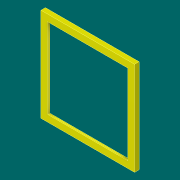
# Autodesk Inventor part: mirrorFrontFrame
Saved by Autodesk Inventor 2016 (Build 200138000, 138)
## iProperties
Created: 2015-10-27
Part Number: mirrorFrontFrame
Material: ABS Plastic
Document SubType Name: Modeling
Designer: Sawaiz
Density: 1.06 g/cm^3
Appearance: Smooth - Yellow
Author: Sawaiz
Autodesk Inventor part; units mm, degrees
ref_plane "YZ Plane" through (0, 0, 0) normal (1, 0, 0) x (0, 1, 0)
ref_plane "XZ Plane" through (0, 0, 0) normal (0, 1, 0) x (-1, 0, 0)
ref_plane "XY Plane" through (0, 0, 0) normal (0, 0, 1) x (1, 0, 0)
sketch "Sketch1" plane through (0, 0, 0) normal (1, 0, 0) x (0, 1, 0)
  line L0 (-66.675, -66.675) -> (66.675, -66.675)
  line L1 (66.675, -66.675) -> (66.675, 66.675)
  line L2 (66.675, 66.675) -> (-66.675, 66.675)
  line L3 (-66.675, 66.675) -> (-66.675, -66.675)
  line L4 (-66.675, -66.675) -> (66.675, 66.675) construction
  line L5 (66.675, -66.675) -> (-66.675, 66.675) construction
  point P0 (0, 0)
  dimension "d0" = 133.35
  dimension "d1" = 133.35
  constraints: 12 end point, 2 midpoint, 2 parallel, 1 horizontal, 1 perpendicular
  measures "d0" distance of L2.end L1.end
  measures "d1" distance of L1.end L0.end
extrude "Extrusion1" add sketch "Sketch1" along normal blind 6.35
sketch "Sketch2" plane through (0, 0, 0) normal (-1, 0, 0) x (0, 0, 1)
  line L0 (60.325, -60.325) -> (-60.325, -60.325)
  line L1 (-60.325, -60.325) -> (-60.325, 60.325)
  line L2 (-60.325, 60.325) -> (60.325, 60.325)
  line L3 (60.325, 60.325) -> (60.325, -60.325)
  line L4 (60.325, -60.325) -> (-60.325, 60.325) construction
  line L5 (-60.325, -60.325) -> (60.325, 60.325) construction
  line L6 (-66.675, -66.675) -> (-66.675, 66.675) projected
  line L7 (66.675, -66.675) -> (-66.675, -66.675) projected
  line L8 (66.675, 66.675) -> (66.675, -66.675) projected
  line L9 (-66.675, 66.675) -> (66.675, 66.675) projected
  line L10 (66.675, 66.675) -> (-66.675, -66.675)
  line L11 (66.675, -66.675) -> (-66.675, -66.675) projected
  line L12 (-66.675, 66.675) -> (66.675, -66.675)
  point P0 (0, 0)
  point P1 (0, 0)
  point P2 (0, 0)
  dimension "d4" = 120.65
  dimension "d5" = 120.65
  constraints: 16 end point, 6 midpoint, 2 parallel, 1 horizontal, 1 perpendicular
  measures "d4" distance of L1.end L2.end
  measures "d5" distance of L0.end L1.end
extrude "Extrusion2" cut sketch "Sketch2" against normal blind 4.7625 contours L12 L10 L3 | L0 L10 L12 | L1 L12 L10 | L10 L12 L2
sketch "Sketch3" plane through (4.7625, 0, 0) normal (-1, 0, 0) x (0, 0, 1)
  line L0 (57.15, -57.15) -> (-57.15, -57.15)
  line L1 (-57.15, -57.15) -> (-57.15, 57.15)
  line L2 (-57.15, 57.15) -> (57.15, 57.15)
  line L3 (57.15, 57.15) -> (57.15, -57.15)
  line L4 (57.15, -57.15) -> (-57.15, 57.15) construction
  line L5 (-57.15, -57.15) -> (57.15, 57.15) construction
  point P0 (0, 0)
  dimension "d8" = 114.3
  dimension "d9" = 114.3
  constraints: 12 end point, 2 midpoint, 2 parallel, 1 horizontal, 1 perpendicular
  measures "d8" distance of L1.end L2.end
  measures "d9" distance of L0.end L1.end
extrude "Extrusion3" cut sketch "Sketch3" against normal through all
equation "\"d0\" = width + internalAcrylicThickness"
equation "\"d1\" = height + internalAcrylicThickness"
equation "\"d2\" = internalAcrylicThickness"
equation "\"d4\" = height - internalAcrylicThickness"
equation "\"d5\" = width - internalAcrylicThickness"
equation "\"d8\" = -internalAcrylicThickness + height - 2 * mirrorThickness"
equation "\"d9\" = -internalAcrylicThickness + width - 2 * mirrorThickness"
equation "\"frameAcrylicThickness\" = 9.525"
equation "\"internalAcrylicThickness\" = 6.35"
equation "\"height\" = 127"
equation "\"width\" = 127"
equation "\"depth\" = 273.05"
equation "\"mirrorAngle\" = 5deg"
equation "\"detectorWidth\" = 52"
equation "\"detectorHeight\" = 52"
equation "\"mirrorThickness\" = 3.175"
equation "\"fresnelThickness\" = 0.1"
equation "\"focalLength\" = 76.2"
equation "\"ior\" = 1.49"
equation "\"centerThickness\" = 1.524"
equation "\"fresnelAngle\" = 90deg"
equation "\"fresnelEffectiveDiameter\" = 152.4"
equation "\"oRingWidth\" = 1.5875"
equation "\"sensorHolderDepth\" = 19.05"
equation "\"aerogelClearence\" = 3.175"
equation "\"backplanePCBWidth\" = 76.2"
equation "\"backplanePCBHeight\" = 76.2"
equation "\"backplaneHoleOffsett\" = 6.35"
equation "\"backplanePostionOffsett\" = 12.7"
equation "\"moduleSlotClearence\" = 0.79375"
body "Solid1"
